Autodesk Fusion 360 part; units mm, degrees
(part 3 of 3)
  constraint parallel L321 L323
  constraint perpendicular L323 L324
  constraint perpendicular L322 L323
  constraint equal L289 L324
  constraint equal L290 L321
  constraint parallel L326 L328
  constraint perpendicular L327 L328
  constraint perpendicular L325 L328
  constraint collinear L27 L326
  constraint equal L324 L327
  constraint equal L321 L328
  constraint collinear L322 L325
  constraint parallel L330 L332
  constraint perpendicular L331 L332
  constraint perpendicular L329 L332
  constraint collinear L39 L332
  constraint collinear L325 L329
  constraint equal L328 L330
  constraint equal L325 L331
  constraint parallel L334 L336
  constraint perpendicular L335 L336
  constraint perpendicular L333 L336
  constraint equal L330 L336
  constraint equal L329 L333
  constraint collinear L329 L333
  constraint collinear L37 L334
  constraint parallel L350 L352
  constraint perpendicular L349 L352
  constraint perpendicular L351 L352
  constraint parallel L346 L347
  constraint perpendicular L346 L348
  constraint perpendicular L345 L346
  constraint equal L348 L349
  constraint equal L346 L350
  constraint collinear L345 L351
  constraint parallel L342 L343
  constraint perpendicular L341 L343
  constraint perpendicular L343 L344
  constraint collinear L344 L345
  constraint equal L342 L346
  constraint equal L341 L345
  constraint parallel L338 L340
  constraint perpendicular L337 L338
  constraint perpendicular L338 L339
  constraint equal L338 L342
  constraint equal L339 L344
  constraint parallel L366 L368
  constraint perpendicular L365 L368
  constraint perpendicular L367 L368
  constraint parallel L362 L363
  constraint perpendicular L362 L364
  constraint perpendicular L361 L362
  constraint equal L364 L365
  constraint equal L362 L366
  constraint collinear L361 L367
  constraint parallel L358 L359
  constraint perpendicular L357 L359
  constraint perpendicular L359 L360
  constraint collinear L360 L361
  constraint equal L358 L362
  constraint equal L357 L361
  constraint parallel L354 L356
  constraint perpendicular L353 L354
  constraint perpendicular L354 L355
  constraint equal L354 L358
  constraint equal L355 L360
  constraint collinear L355 L360
  constraint collinear L34 L340
  constraint collinear L32 L343
  constraint collinear L47 L347
  constraint collinear L45 L352
  constraint collinear L54 L356
  constraint collinear L349 L353
  constraint collinear L52 L359
  constraint collinear L58 L363
  constraint collinear L56 L368
  constraint equal L333 L337
  constraint equal L336 L338
  constraint collinear L337 L341
  constraint equal L351 L353
  constraint equal L350 L354
  constraint parallel L382 L383
  constraint perpendicular L383 L384
  constraint perpendicular L381 L383
  constraint parallel L377 L379
  constraint perpendicular L377 L380
  constraint perpendicular L377 L378
  constraint equal L380 L384
  constraint equal L377 L382
  constraint collinear L378 L381
  constraint parallel L374 L376
  constraint perpendicular L373 L374
  constraint perpendicular L374 L375
  constraint collinear L375 L378
  constraint equal L376 L377
  constraint equal L373 L378
  constraint parallel L369 L372
  constraint perpendicular L370 L372
  constraint perpendicular L371 L372
  constraint equal L372 L376
  constraint equal L371 L375
  constraint parallel L398 L400
  constraint perpendicular L397 L398
  constraint perpendicular L398 L399
  constraint parallel L394 L396
  constraint perpendicular L393 L394
  constraint perpendicular L394 L395
  constraint equal L393 L397
  constraint equal L394 L400
  constraint collinear L395 L399
  constraint parallel L389 L390
  constraint perpendicular L390 L392
  constraint perpendicular L390 L391
  constraint collinear L391 L395
  constraint equal L389 L394
  constraint equal L392 L395
  constraint parallel L386 L388
  constraint perpendicular L385 L386
  constraint perpendicular L386 L387
  constraint equal L386 L389
  constraint equal L387 L391
  constraint collinear L387 L391
  constraint collinear L384 L385
  constraint collinear L370 L373
  constraint equal L381 L385
  constraint equal L382 L386
  constraint equal L338 L372
  constraint equal L339 L370
  constraint collinear L42 L369
  constraint collinear L40 L374
  constraint collinear L30 L379
  constraint collinear L28 L383
  constraint collinear L50 L388
  constraint collinear L48 L390
  constraint collinear L62 L396
  constraint collinear L60 L398
  constraint parallel L414 L415
  constraint perpendicular L415 L416
  constraint perpendicular L413 L415
  constraint parallel L409 L411
  constraint perpendicular L409 L412
  constraint perpendicular L409 L410
  constraint equal L412 L416
  constraint equal L409 L414
  constraint collinear L410 L413
  constraint parallel L406 L408
  constraint perpendicular L405 L406
  constraint perpendicular L406 L407
  constraint collinear L407 L410
  constraint equal L408 L409
  constraint equal L405 L410
  constraint parallel L401 L404
  constraint perpendicular L402 L404
  constraint perpendicular L403 L404
  constraint equal L404 L408
  constraint equal L403 L407
  constraint parallel L430 L432
  constraint perpendicular L429 L430
  constraint perpendicular L430 L431
  constraint parallel L426 L428
  constraint perpendicular L425 L426
  constraint perpendicular L426 L427
  constraint equal L425 L429
  constraint equal L426 L432
  constraint collinear L427 L431
  constraint parallel L421 L422
  constraint perpendicular L422 L424
  constraint perpendicular L422 L423
  constraint collinear L423 L427
  constraint equal L421 L426
  constraint equal L424 L427
  constraint parallel L418 L420
  constraint perpendicular L417 L418
  constraint perpendicular L418 L419
  constraint equal L418 L421
  constraint equal L419 L423
  constraint collinear L419 L423
  constraint collinear L416 L417
  constraint collinear L402 L405
  constraint equal L413 L417
  constraint equal L414 L418
  constraint parallel L446 L447
  constraint perpendicular L447 L448
  constraint perpendicular L445 L447
  constraint parallel L441 L443
  constraint perpendicular L441 L444
  constraint perpendicular L441 L442
  constraint equal L444 L448
  constraint equal L441 L446
  constraint collinear L442 L445
  constraint parallel L438 L440
  constraint perpendicular L437 L438
  constraint perpendicular L438 L439
  constraint collinear L439 L442
  constraint equal L440 L441
  constraint equal L437 L442
  constraint parallel L433 L436
  constraint perpendicular L434 L436
  constraint perpendicular L435 L436
  constraint equal L436 L440
  constraint equal L435 L439
  constraint parallel L462 L464
  constraint perpendicular L461 L462
  constraint perpendicular L462 L463
  constraint parallel L458 L460
  constraint perpendicular L457 L458
  constraint perpendicular L458 L459
  constraint equal L457 L461
  constraint equal L458 L464
  constraint collinear L459 L463
  constraint parallel L453 L454
  constraint perpendicular L454 L456
  constraint perpendicular L454 L455
  constraint collinear L455 L459
  constraint equal L453 L458
  constraint equal L456 L459
  constraint parallel L450 L452
  constraint perpendicular L449 L450
  constraint perpendicular L450 L451
  constraint equal L450 L453
  constraint equal L451 L455
  constraint collinear L451 L455
  constraint collinear L448 L449
  constraint collinear L434 L437
  constraint equal L445 L449
  constraint equal L446 L450
  constraint parallel L478 L479
  constraint perpendicular L479 L480
  constraint perpendicular L477 L479
  constraint parallel L473 L475
  constraint perpendicular L473 L476
  constraint perpendicular L473 L474
  constraint equal L476 L480
  constraint equal L473 L478
  constraint collinear L474 L477
  constraint parallel L470 L472
  constraint perpendicular L469 L470
  constraint perpendicular L470 L471
  constraint collinear L471 L474
  constraint equal L472 L473
  constraint equal L469 L474
  constraint parallel L465 L468
  constraint perpendicular L466 L468
  constraint perpendicular L467 L468
  constraint equal L468 L472
  constraint equal L467 L471
  constraint parallel L494 L496
  constraint perpendicular L493 L494
  constraint perpendicular L494 L495
  constraint parallel L490 L492
  constraint perpendicular L489 L490
  constraint perpendicular L490 L491
  constraint equal L489 L493
  constraint equal L490 L496
  constraint collinear L491 L495
  constraint parallel L485 L486
  constraint perpendicular L486 L488
  constraint perpendicular L486 L487
  constraint collinear L487 L491
  constraint equal L485 L490
  constraint equal L488 L491
  constraint parallel L482 L484
  constraint perpendicular L481 L482
  constraint perpendicular L482 L483
  constraint equal L482 L485
  constraint equal L483 L487
  constraint collinear L483 L487
  constraint collinear L480 L481
  constraint collinear L466 L469
  constraint equal L477 L481
  constraint equal L478 L482
  constraint parallel L510 L511
  constraint perpendicular L511 L512
  constraint perpendicular L509 L511
  constraint parallel L505 L507
  constraint perpendicular L505 L508
  constraint perpendicular L505 L506
  constraint equal L508 L512
  constraint equal L505 L510
  constraint collinear L506 L509
  constraint parallel L502 L504
  constraint perpendicular L501 L502
  constraint perpendicular L502 L503
  constraint collinear L503 L506
  constraint equal L504 L505
  constraint equal L501 L506
  constraint parallel L497 L500
  constraint perpendicular L498 L500
  constraint perpendicular L499 L500
  constraint equal L500 L504
  constraint equal L499 L503
  constraint parallel L526 L528
  constraint perpendicular L525 L526
  constraint perpendicular L526 L527
  constraint parallel L522 L524
  constraint perpendicular L521 L522
  constraint perpendicular L522 L523
  constraint equal L521 L525
  constraint equal L522 L528
  constraint collinear L523 L527
  constraint parallel L517 L518
  constraint perpendicular L518 L520
  constraint perpendicular L518 L519
  constraint collinear L519 L523
  constraint equal L517 L522
  constraint equal L520 L523
  constraint parallel L514 L516
  constraint perpendicular L513 L514
  constraint perpendicular L514 L515
  constraint equal L514 L517
  constraint equal L515 L519
  constraint collinear L515 L519
  constraint collinear L512 L513
  constraint collinear L498 L501
  constraint equal L509 L513
  constraint equal L510 L514
  constraint collinear L17 L401
  constraint equal L372 L404
  constraint equal L371 L403
  constraint equal L402 L434
  constraint equal L404 L436
  constraint equal L436 L468
  constraint equal L435 L466
  constraint equal L467 L498
  constraint equal L468 L500
  constraint collinear L19 L406
  constraint collinear L10 L411
  constraint collinear L8 L415
  constraint collinear L3 L420
  constraint collinear L1 L422
  constraint collinear L221 L428
  constraint collinear L223 L430
  constraint collinear L187 L462
  constraint collinear L185 L460
  constraint collinear L7 L454
  constraint collinear L5 L452
  constraint collinear L183 L447
  constraint collinear L181 L443
  constraint collinear L13 L438
  constraint collinear L15 L433
  constraint collinear L195 L465
  constraint collinear L193 L470
  constraint collinear L205 L475
  constraint collinear L207 L479
  constraint collinear L214 L484
  constraint collinear L212 L486
  constraint collinear L176 L492
  constraint collinear L178 L494
  constraint collinear L197 L526
  constraint collinear L199 L524
  constraint collinear L191 L518
  constraint collinear L189 L516
  constraint collinear L211 L511
  constraint collinear L209 L507
  constraint collinear L203 L502
  constraint collinear L201 L497
  constraint parallel L533 L535
  constraint perpendicular L533 L536
  constraint perpendicular L533 L534
  constraint parallel L529 L532
  constraint perpendicular L529 L530
  constraint perpendicular L529 L531
  constraint equal L530 L536
  constraint equal L529 L535
  constraint collinear L531 L534
  constraint parallel L541 L543
  constraint perpendicular L541 L544
  constraint perpendicular L541 L542
  constraint parallel L537 L540
  constraint perpendicular L537 L538
  constraint perpendicular L537 L539
  constraint equal L538 L544
  constraint equal L537 L543
  constraint collinear L539 L542
  constraint parallel L549 L551
  constraint perpendicular L549 L552
  constraint perpendicular L549 L550
  constraint parallel L545 L548
  constraint perpendicular L545 L546
  constraint perpendicular L545 L547
  constraint equal L546 L552
  constraint equal L545 L551
  constraint collinear L547 L550
  constraint collinear L525 L546
  constraint collinear L216 L548
  constraint collinear L218 L549
  constraint equal L528 L545
  constraint equal L527 L547
  constraint collinear L20 L540
  constraint collinear L22 L541
  constraint collinear L493 L538
  constraint equal L496 L537
  constraint equal L495 L539
  constraint collinear L225 L532
  constraint collinear L461 L530
  constraint collinear L227 L533
  constraint equal L463 L531
  constraint equal L464 L529
  constraint parallel L557 L559
  constraint perpendicular L557 L560
  constraint perpendicular L557 L558
  constraint parallel L553 L556
  constraint perpendicular L553 L554
  constraint perpendicular L553 L555
  constraint equal L554 L560
  constraint equal L553 L559
  constraint collinear L555 L558
  constraint collinear L102 L556
  constraint collinear L100 L557
  constraint equal L432 L553
  constraint equal L399 L555
  constraint perpendicular L119 L561
  constraint perpendicular L114 L562
  constraint coincident L109 L563.start
  constraint perpendicular L109 L563
  constraint perpendicular L108 L564
  constraint coincident L109 L565.end
  constraint perpendicular L109 L565
  constraint perpendicular L126 L567
  constraint coincident L137 L569.start
  constraint perpendicular L137 L569
  constraint perpendicular L569 L570
  constraint coincident L137 L571.end
  constraint perpendicular L137 L571
  constraint equal L565 L569
  constraint equal L564 L570
  constraint perpendicular L168 L573
  constraint perpendicular L173 L574
  constraint perpendicular L155 L576
  constraint coincident L142 L577.start
  constraint perpendicular L142 L577
  constraint perpendicular L577 L578
  constraint coincident L142 L579.end
  constraint perpendicular L142 L579
  constraint equal L570 L578
  constraint equal L571 L577
  constraint coincident L150 L581.start
  constraint perpendicular L150 L581
  constraint perpendicular L581 L582
  constraint coincident L150 L583.end
  constraint perpendicular L150 L583
  constraint equal L577 L583
  constraint equal L578 L582
  constraint perpendicular L82 L586
  constraint perpendicular L94 L587
  constraint coincident L69 L589.start
  constraint perpendicular L69 L589
  constraint perpendicular L589 L590
  constraint coincident L69 L591.end
  constraint perpendicular L69 L591
  constraint equal L578 L590
  constraint equal L579 L591
  constraint coincident L77 L593.start
  constraint perpendicular L77 L593
  constraint perpendicular L593 L594
  constraint coincident L77 L595.end
  constraint perpendicular L77 L595
  constraint equal L578 L594
  constraint equal L591 L595
  constraint collinear L598 L601
  constraint horizontal L602
  constraint vertical L603
  constraint collinear L603 L605
  constraint horizontal L597
  constraint horizontal L607
  constraint vertical L608
  constraint horizontal L609
  constraint vertical L610
  constraint horizontal L611
  constraint vertical L612
  constraint horizontal L613
  constraint vertical L614
  constraint collinear L607 L615
  constraint collinear L611 L616
  constraint equal L609 L613
  constraint equal L608 L614
  constraint equal L589 L610
  constraint equal L590 L609
  constraint perpendicular L568 L617
  constraint coincident L132 L618.end
  constraint perpendicular L125 L618
  constraint coincident L114 L619.end
  constraint perpendicular L114 L619
  constraint perpendicular L619 L620
  constraint collinear L121 L619
  constraint collinear L562 L567
  constraint collinear L120 L561
  constraint collinear L126 L568
  constraint parallel L623 L624
  constraint perpendicular L621 L623
  constraint perpendicular L622 L623
  constraint collinear L105 L623
  constraint equal L560 L622
  constraint equal L559 L624
  constraint parallel L627 L628
  constraint perpendicular L625 L627
  constraint perpendicular L626 L627
  constraint collinear L146 L627
  constraint equal L624 L628
  constraint equal L621 L626
  constraint coincident L173 L629.end
  constraint perpendicular L574 L629
  constraint coincident L155 L630.end
  constraint perpendicular L155 L630
  constraint perpendicular L576 L631
  constraint collinear L166 L630
  constraint collinear L574 L576
  constraint collinear L161 L575
  constraint collinear L167 L573
  constraint coincident L64 L633.end
  constraint perpendicular L587 L633
  constraint coincident L82 L634.end
  constraint perpendicular L82 L634
  constraint perpendicular L586 L635
  constraint perpendicular L585 L636
  constraint collinear L93 L634
  constraint collinear L586 L587
  constraint collinear L88 L585
  constraint collinear L94 L588
  constraint parallel L639 L640
  constraint perpendicular L637 L639
  constraint perpendicular L638 L639
  constraint collinear L73 L639
  constraint equal L366 L640
  constraint equal L365 L638
  constraint coincident L600 L641.end
  constraint perpendicular L597 L641
  constraint coincident L604 L642.end
  constraint perpendicular L604 L642
  constraint perpendicular L602 L643
  constraint perpendicular L598 L644
  constraint collinear L597 L602
  constraint collinear L642 L645
  constraint horizontal L647
  constraint vertical L648
  constraint horizontal L646
  constraint vertical L649
  constraint collinear L646 L650
  constraint collinear L283 L649
  constraint equal L281 L648
  constraint collinear L281 L648
  measures "d504" distance of L237 L239
  measures "d508" distance of L243 L248
  measures "d510" distance of L246 L249
  measures "d511" distance of L17 L231
  measures "d514" distance of L229 L233
  measures "d515" distance of L228 L232
  measures "d516" distance of L230 L231
  measures "d517" distance of L238 L240
  measures "d518" distance of L238 L246
  measures "d519" distance of L244 L247
  measures "d520" distance of L245 L251
  measures "d563" distance of L254 L256
  measures "d564" distance of L252.end L253.end
  measures "d565" distance of L253 L255
  measures "d566" distance of L257 L258
  measures "d567" distance of L254 L263
  measures "d568" distance of L271 L275
  measures "d569" distance of L270 L276
  measures "d570" distance of L271.end L281.end
  measures "d571" distance of L281.end L289.end
  measures "d572" distance of L296 L309
  measures "d614" distance of L24 L324
  measures "d638" distance of L33 L339
  measures "d639" distance of L43 L370
  measures "d640" distance of L18 L402
  measures "d641" distance of L12 L434
  measures "d642" distance of L192 L466
  measures "d643" distance of L202 L498
  measures "d644" distance of L103 L554
  measures "d674" distance of L563.end L564.end
  measures "d676" distance of L108.end L565
  measures "d678" distance of L564 L566
  measures "d679" distance of L137.end L569.start
  measures "d680" distance of L141 L579
  measures "d681" distance of L149 L583
  measures "d682" distance of L68 L589
  measures "d683" distance of L78 L593
  measures "d684" distance of L610 L615.end
  measures "d685" distance of L612 L616.start
  measures "d687" distance of L115 L562
  measures "d688" distance of L562 L617
  measures "d689" distance of L106 L622
  measures "d690" distance of L145 L625.start
  measures "d691" distance of L576 L632
  measures "d692" distance of L156 L576
  measures "d693" distance of L83 L586
  measures "d694" distance of L586 L636
  measures "d695" distance of L72 L637
  measures "d696" distance of L597 L599
  measures "d697" distance of L597 L644
extrude "Rahmen Rechts" add sketch "Skizze4" along normal up to surface separate body contours L228 L229 A0 L230 A1 L237 L238 A2 end surface through (0, 80, 16.2816) normal (0, 0.043619, -0.999048) offset 0 makes body 3
extrude "Rahmen Mitte" add sketch "Skizze4" along normal up to surface separate body contours L238 L247 L248 L251 end surface through (0, 80, 16.2816) normal (0, 0.043619, -0.999048) offset 0 makes body 4
fillet "Abrundung1" radius 2 7 edges at (-104.3906, 28.0489, 0) (-163.9894, 43.7866, 0) (-62.3093, 1.7662, 0) (-41.6839, 0, 0) (-176.2508, 102.7417, 0) (-100.1502, 146.1161, 0) (-32.4236, 134.2339, 0) on bodies 1 2
fillet "Abrundung1" radius 2 2 edges at (0, 0, 0) (0, 134.175, 0) on bodies 1 2
ref_plane "Arbeitsebene2" through (0, 0, 10.7) normal (0, 0, 1) x (1, 0, 0)
sketch "Skizze6" plane through (0, 0, 10.7) normal (0, 0, 1) x (1, 0, 0)
  line L0 (-163.5373, 153.5359) -> (-33.425, 130.5936)
  line L1 (-164.3485, 154.6944) -> (-32.425, 131.4327)
  line L2 (-163.5373, 153.5359) -> (-181.6767, 50.6624)
  line L3 (-182.8351, 49.8513) -> (-164.3485, 154.6944)
  line L4 (-181.6767, 50.6624) -> (-141.3734, 43.5559)
  line L5 (-141.5471, 42.5711) -> (-182.8351, 49.8513)
  line L6 (-141.3734, 43.5559) -> (-141.5471, 42.5711) construction
  line L7 (-52.2928, 3.7) -> (-33.425, 3.7)
  arc A0 (-68.7394, 9.6861) -> (-141.3734, 43.5559) centre (-168.2583, -108.916) ccw
  arc A1 (-68.7394, 9.6861) -> (-52.2928, 3.7) centre (-52.2928, 29.2863) ccw
  line L8 (0, 130.475) -> (0, 128.475) construction
  line L9 (0, 128.475) -> (-11, 128.475)
  line L10 (-11, 128.475) -> (-11, 130.475)
  line L11 (0, 128.475) -> (11, 128.475)
  line L12 (11, 128.475) -> (11, 130.475)
  line L13 (-52.2928, 3.7) -> (-52.2928, 2.7) construction
  line L14 (-32.425, 2.7) -> (-52.2928, 2.7) construction
  line L15 (-68.7394, 9.6861) -> (-69.3822, 8.92) construction
  line L16 (-58.4402, 21.9601) -> (-59.4205, 20.7919) construction
  line L17 (-33.425, 3.7) -> (-33.425, 130.5936)
  line L18 (-32.425, 131.4327) -> (-32.425, 2.7)
  line L19 (28.725, 3.7) -> (-28.725, 3.7)
  line L20 (-28.725, 3.7) -> (-28.725, 130.475)
  line L21 (-28.725, 130.475) -> (28.725, 130.475)
  line L22 (28.725, 130.475) -> (28.725, 3.7)
  line L23 (29.725, 131.475) -> (29.725, 2.7)
  line L24 (29.725, 2.7) -> (-29.725, 2.7)
  line L25 (-29.725, 2.7) -> (-29.725, 131.475)
  line L26 (-29.725, 131.475) -> (29.725, 131.475)
  line L27 (0, 1.75) -> (0, 22.5)
  point P0 (-52.2928, 2.7)
  point P1 (-69.3822, 8.92)
  dimension "d489" = 2
  dimension "d490" = 11
  dimension "d491" = 11
  dimension "d525" = 1
  dimension "d526" = 1
  dimension "d527" = 1
  dimension "d528" = 1
  dimension "d529" = 1
  dimension "d530" = 1
  dimension "d531" = 1
  dimension "d532" = 1
  dimension "d533" = 1
  constraint parallel L0 L1
  constraint perpendicular L0 L2
  constraint perpendicular L2 L4
  constraint coincident L5.start L6.end
  constraint perpendicular L4 L6
  constraint tangent L4 A0
  constraint tangent A0 A1
  constraint vertical L8
  constraint perpendicular L8 L9
  constraint perpendicular L9 L10
  constraint perpendicular L8 L11
  constraint perpendicular L11 L12
  constraint horizontal L7
  constraint perpendicular L7 L13
  constraint coincident P0 L13.end
  constraint tangent L7 A1
  constraint coincident P1 L15.end
  constraint collinear L15 L16
  constraint parallel L17 L18
  constraint horizontal L19
  constraint vertical L20
  constraint horizontal L21
  constraint vertical L22
  constraint coincident L12.end L21
  constraint coincident L8.start L21
  constraint coincident L10.end L21
  constraint collinear L8 L27
  measures "d489" distance of L8.start L8.end
  measures "d490" distance of L8.end L9.end
  measures "d491" distance of L8.end L11.end
  measures "d525" distance of L7 L14
  measures "d526" distance of L4 L5
  measures "d527" distance of L2 L3
  measures "d528" distance of L0 L1
  measures "d529" distance of L17 L18
  measures "d530" distance of L22 L23
  measures "d531" distance of L19 L24
  measures "d532" distance of L20 L25
  measures "d533" distance of L21 L26
extrude "Bodenplatte Rechts" add sketch "Skizze6" along normal up to surface separate body contours L0 L2 L4 L7 A0 A1 L17 end surface through (0, 80, 16.2816) normal (0, 0.043619, -0.999048) offset 0 makes body 5
extrude "Bodenplatte Mitte" add sketch "Skizze6" along normal up to surface separate body contours L9 L10 L11 L12 L19 L20 L21 L22 | L9 L10 L11 L12 L21 end surface through (0, 80, 16.2816) normal (0, 0.043619, -0.999048) offset 0 makes body 6
extrude "Lasche an Bodenplatte" add sketch "Skizze6" against normal blind 6 contours L9 L10 L11 L12 L21 bodies 6
ref_plane "Arbeitsebene3" through (-107.5508, 78.7357, 13.5239) normal (0, -0.043619, 0.999048) x (1, 0, 0)
sketch "Skizze7" plane through (0, 78.9574, 13.5335) normal (0, -0.043619, 0.999048) x (1, 0, 0)
  line L0 (11, 49.6846) -> (-11, 49.6846)
  line L1 (0, -77.7242) -> (0, -56.994)
  line L2 (11, 49.6846) -> (11, -2.3154)
  line L3 (11, -2.3154) -> (-11, -2.3154)
  line L4 (-11, -2.3154) -> (-11, 49.6846)
  circle A0 centre (-5.7, 0.1846) radius 0.75
  circle A1 centre (5.7, 0.1846) radius 0.75
  circle A2 centre (5.7, 47.1846) radius 0.75
  circle A3 centre (-5.7, 47.1846) radius 0.75
  line L5 (28.725, 51.6846) -> (-28.725, 51.6846)
  line L6 (-13, -2.3154) -> (-13, 51.6846)
  line L7 (-13, 51.6846) -> (-28.725, 51.6846)
  line L8 (-28.725, 51.6846) -> (-28.725, -75.3094)
  line L9 (-28.725, -75.3094) -> (28.725, -75.3094)
  line L10 (28.725, -75.3094) -> (28.725, 51.6846)
  line L11 (28.725, 51.6846) -> (13, 51.6846)
  line L12 (13, 51.6846) -> (13, -2.3154)
  line L13 (11, -4.3154) -> (-11, -4.3154)
  arc A4 (11, -4.3154) -> (13, -2.3154) centre (11, -2.3154) ccw
  arc A5 (-13, -2.3154) -> (-11, -4.3154) centre (-11, -2.3154) ccw
  line L14 (-28.725, -75.3094) -> (-28.725, 51.345)
  line L15 (28.725, 51.345) -> (28.725, -75.3094)
  line L16 (28.725, -75.3094) -> (-28.725, -75.3094)
  line L17 (11, 49.6846) -> (13, 49.6846)
  line L18 (-11, 49.6846) -> (-13, 49.6846)
  dimension "d458" = 52
  dimension "d460" = 1.5
  dimension "d461" = 1.5
  dimension "d462" = 2.5
  dimension "d463" = 2.5
  dimension "d464" = 5.3
  dimension "d465" = 5.3
  dimension "d466" = 11.4
  dimension "d467" = 1.5
  dimension "d468" = 1.5
  dimension "d469" = 2.5
  dimension "d470" = 2.5
  dimension "d471" = 5.3
  dimension "d472" = 5.3
  dimension "d473" = 11.4
  dimension "d536" = 2
  dimension "d537" = 11
  dimension "d538" = 11
  dimension "d704" = 2
  constraint horizontal L0
  constraint perpendicular L0 L2
  constraint perpendicular L2 L3
  constraint perpendicular L0 L4
  constraint perpendicular L5 L6
  constraint perpendicular L6 L7
  constraint perpendicular L8 L9
  constraint perpendicular L5 L10
  constraint parallel L5 L11
  constraint perpendicular L3 L12
  constraint perpendicular L4 L13
  constraint coincident L2.end L3.start
  constraint coincident L3 L6.start
  constraint coincident L4 L13.end
  constraint coincident L2 L13.start
  constraint coincident L3 L12.end
  constraint tangent L6 A5
  constraint tangent L13 A5
  constraint collinear L5 L7
  constraint collinear L5 L11
  constraint collinear L8 L14
  constraint collinear L10 L15
  constraint collinear L9 L16
  constraint coincident L12 L17.end
  constraint perpendicular L12 L17
  constraint coincident L6 L18.end
  constraint perpendicular L6 L18
  measures "d458" distance of L0.start L2.end
  measures "d460" diameter of A0
  measures "d461" diameter of A1
  measures "d462" distance of L3 A1.centre
  measures "d463" distance of L3 A0.centre
  measures "d464" distance of L4 A0.centre
  measures "d465" distance of L2 A1.centre
  measures "d466" distance of A0.centre A1.centre
  measures "d467" diameter of A2
  measures "d468" diameter of A3
  measures "d469" distance of L0 A3.centre
  measures "d470" distance of L0 A2.centre
  measures "d471" distance of L4 A3.centre
  measures "d472" distance of L2 A2.centre
  measures "d473" distance of A2.centre A3.centre
  measures "d536" distance of L0 L5
  measures "d537" distance of L1 L2
  measures "d538" distance of L1 L4
  measures "d704" distance of L3 L13
extrude "Ausschnitt Controller (1)" cut sketch "Skizze7" against normal through all contours L0 L2 L3 L4 | L2 L3 L4 L6 L12 L13 A4 A5 L17 L18 | L5 L6 L7 L8 L9 L10 L11 L12 L13 A4 A5 L14 L15 L16 | A0 | A1 | A2 | A3 bodies 6
extrude "Stifte Controller" add sketch "Skizze7" against normal blind 1.5 contours L2 L3 L4 L6 L12 L13 A4 A5 L17 L18 | A0 | A1 | A2 | A3 bodies 6
extrude "Extrusion27" add sketch "Skizze1" along normal up to surface from surface at 10.7 contours A3 | A4 | A5 | A6 | A7 | A8 | A9 | A10 | A11 | A12 | A13 | A14 | A39 | A40 | A41 | A42 | A43 | A44 | A57 | A58 | A59 | A60 | A61 | A62 end surface through (0, 78.9574, 13.5335) normal (0, 0.043619, -0.999048) offset 0 bodies 6
sketch "Skizze8" plane through (0, 129.0342, 5.6338) normal (0, -0.999048, -0.043619) x (1, 0, 0)
  line L0 (11, 10.0766) -> (-11, 10.0766)
  line L1 (4.5, 5.0766) -> (-4.5, 5.0766)
  line L2 (-4.5, 5.0766) -> (-4.5, 9.0766)
  line L3 (-4.5, 9.0766) -> (4.5, 9.0766)
  line L4 (4.5, 9.0766) -> (4.5, 5.0766)
  line L5 (7, 2.0766) -> (-7, 2.0766)
  line L6 (-7, 2.0766) -> (-7, 13.0766)
  line L7 (7, 2.0766) -> (7, 13.0766)
  line L8 (7, 13.0766) -> (-7, 13.0766)
  line L9 (-11, -0.9346) -> (11, -0.9346)
  line L10 (11, -0.9346) -> (11, 5.0711)
  line L11 (-11, 5.0711) -> (-11, -0.9346)
  line L12 (11, 5.0711) -> (13, 5.0711)
  line L13 (13, 5.0711) -> (13, 8.5766)
  line L14 (-13, 8.5766) -> (-13, 5.0711)
  line L15 (-13, 5.0711) -> (-11, 5.0711)
  line L16 (-11, 8.5766) -> (-13, 8.5766)
  line L17 (13, 8.5766) -> (11, 8.5766)
  line L18 (11, 8.5766) -> (11, 10.0766)
  line L19 (-11, 10.0766) -> (-11, 8.5766)
  line L20 (11, 5.0711) -> (11, 8.5766)
  line L21 (-11, 5.0711) -> (-11, 8.5766)
  line L22 (13, 5.0711) -> (13, 4.0711)
  line L23 (13, 4.0711) -> (11, 4.0711)
  line L24 (-13, 5.0711) -> (-13, 4.0711)
  line L25 (-13, 4.0711) -> (-11, 4.0711)
  dimension "d477" = 5
  dimension "d478" = 1
  dimension "d485" = 8
  dimension "d486" = 14
  dimension "d487" = 11
  dimension "d542" = 2.5
  dimension "d576" = 6.5
  dimension "d714" = 9
  dimension "d715" = 4
  dimension "d716" = 2.5
  dimension "d717" = 1
  dimension "d718" = 1
  constraint horizontal L1
  constraint vertical L2
  constraint horizontal L3
  constraint vertical L4
  constraint horizontal L5
  constraint perpendicular L0 L6
  constraint perpendicular L0 L7
  constraint horizontal L8
  constraint coincident L10.end L12.start
  constraint coincident L17.end L18.start
  constraint coincident L11.start L15.end
  constraint coincident L16.start L19.end
  constraint coincident L12.end L13.start
  constraint perpendicular L12 L22
  constraint coincident L10 L23.end
  constraint perpendicular L10 L23
  constraint coincident L14.end L15.start
  constraint perpendicular L15 L24
  constraint coincident L11 L25.end
  constraint perpendicular L11 L25
  measures "d477" distance of L0 L1
  measures "d478" distance of L0 L3
  measures "d485" distance of L0 L5
  measures "d486" distance of L5.start L5.end
  measures "d487" distance of L5 L8
  measures "d542" distance of L2 L6
  measures "d576" horizontal distance of L1.end L9.start
  measures "d714" distance of L1.start L1.end
  measures "d715" distance of L6 L11
  measures "d716" distance of L4 L7
  measures "d717" distance of L12.end L22.end
  measures "d718" distance of L14.end L24.end
extrude "Öffnung in Grundplatte" cut sketch "Skizze8" against normal through all contours L12 L13 L17 L20 | L10 L12 L22 L23 | L14 L15 L16 L21 | L11 L15 L24 L25 | L1 L2 L3 L4 bodies 6
extrude "Öffnug in Rahmen" cut sketch "Skizze8" against normal through all contours L0 L5 L6 L7 | L0 L6 L7 L8 | L1 L2 L3 L4 bodies 4
extrude "Stehhülsen" add sketch "Skizze1" along normal blind 10.7 contours A3 | A4 | A5 | A6 | A7 | A8 | A9 | A10 | A11 | A12 | A13 | A14 | A15 | A16 | A17 | A18 | A19 | A20 | A21 | A22 | A23 | A24 | A25 | A26 | A27 | A28 | A29 | A30 | A31 | A32 | A33 | A34 | A35 | A36 | A37 | A38 bodies 1 2 3 4
extrude "Bohrungen" cut sketch "Skizze1" along normal through all contours A3 | A5 | A7 | A9 | A11 | A13 | A15 | A17 | A19 | A21 | A23 | A25 | A27 | A29 | A31 | A33 | A35 | A37 | A39 | A40 | A41 | A42 | A43 | A44 | A45 | A46 | A47 | A48 | A49 | A50 | A51 | A52 | A53 | A54 | A55 | A56 bodies 5 6
extrude "Senkungen" cut sketch "Skizze1" along normal through all from surface at 12.2 contours A4 | A6 | A8 | A10 | A12 | A14 | A16 | A18 | A20 | A22 | A24 | A26 | A28 | A30 | A32 | A34 | A36 | A38 bodies 5 6
extrude "Kerben" cut sketch "Skizze4" against normal blind 1.4 contours L3 L417 L418 L419 L420 | L1 L421 L422 L423 L424 | L7 L453 L454 L455 L456 | L5 L449 L450 L451 L452 | L8 L413 L414 L415 L416 | L10 L409 L410 L411 L412 | L15 L433 L434 L435 L436 | L13 L437 L438 L439 L440 | L19 L405 L406 L407 L408 | L17 L401 L402 L403 L404 | L20 L537 L538 L539 L540 | L22 L541 L542 L543 L544 | L27 L325 L326 L327 L328 | L25 L321 L322 L323 L324 | L28 L381 L382 L383 L384 | L30 L377 L378 L379 L380 | L32 L341 L342 L343 L344 | L34 L337 L338 L339 L340 | L39 L329 L330 L331 L332 | L37 L333 L334 L335 L336 | L40 L373 L374 L375 L376 | L42 L369 L370 L371 L372 | L47 L345 L346 L347 L348 | L45 L349 L350 L351 L352 | L48 L389 L390 L391 L392 | L50 L385 L386 L387 L388 | L52 L357 L358 L359 L360 | L54 L353 L354 L355 L356 | L56 L365 L366 L367 L368 | L58 L361 L362 L363 L364 | L60 L397 L398 L399 L400 | L62 L393 L394 L395 L396 | L83 L84 L85 L86 L87 L88 L89 L90 L91 L92 L93 L94 L95 L96 L97 L98 L99 L585 L586 L587 L588 L633 L634 L635 L636 | L69 L589 L590 L591 L592 | L77 L593 L594 L595 L596 | L73 L637 L638 L639 L640 | L100 L557 L558 L559 L560 | L102 L553 L554 L555 L556 | L105 L621 L622 L623 L624 | L137 L569 L570 L571 L572 | L109 L563 L564 L565 L566 | L115 L116 L117 L118 L119 L120 L121 L122 L123 L124 L125 L126 L127 L128 L129 L130 L131 L561 L562 L567 L568 L617 L618 L619 L620 | L142 L577 L578 L579 L580 | L156 L157 L158 L159 L160 L161 L162 L163 L164 L165 L166 L167 L168 L169 L170 L171 L172 L573 L574 L575 L576 L629 L630 L631 L632 | L146 L625 L626 L627 L628 | L150 L581 L582 L583 L584 | L176 L489 L490 L491 L492 | L178 L493 L494 L495 L496 | L183 L445 L446 L447 L448 | L181 L441 L442 L443 L444 | L187 L461 L462 L463 L464 | L185 L457 L458 L459 L460 | L191 L517 L518 L519 L520 | L189 L513 L514 L515 L516 | L195 L465 L466 L467 L468 | L193 L469 L470 L471 L472 | L199 L521 L522 L523 L524 | L197 L525 L526 L527 L528 | L203 L501 L502 L503 L504 | L201 L497 L498 L499 L500 | L207 L477 L478 L479 L480 | L205 L473 L474 L475 L476 | L211 L509 L510 L511 L512 | L209 L505 L506 L507 L508 | L212 L485 L486 L487 L488 | L214 L481 L482 L483 L484 | L216 L545 L546 L547 L548 | L218 L549 L550 L551 L552 | L223 L429 L430 L431 L432 | L221 L425 L426 L427 L428 | L227 L533 L534 L535 L536 | L225 L529 L530 L531 L532 | L252 L253 L254 L257 | L258 L259 L260 L261 | L262 L263 L264 L265 | L266 L267 L268 L269 | L270 L271 L272 L273 L274 | L276 L277 L278 L279 | L280 L281 L282 L283 | L284 L285 L286 L287 | L288 L289 L290 L291 | L292 L293 L294 L295 | L296 L297 L298 L299 L300 | L301 L302 L303 L304 | L305 L306 L307 L308 | L309 L310 L311 L312 | L313 L314 L315 L316 | L317 L318 L319 L320 | L597 L598 L600 L602 L603 L604 L641 L642 L643 L644 L645 | L607 L608 L609 L610 L615 | L611 L612 L613 L614 L616 | L646 L647 L648 L649 L650 bodies 1 2
sketch "Skizze9" plane through (-32.425, 0, 0) normal (-1, 0, 0) x (0, -1, 0)
  line L0 (-2.7, 12.9066) -> (-131.4327, 18.5272)
  line L1 (-131.4327, 18.5272) -> (-131.4327, 2.7)
  line L2 (-131.4327, 2.7) -> (-2.7, 2.7)
  line L3 (-2.7, 2.7) -> (-2.7, 12.9066)
  circle A0 centre (-104.8827, 10.034) radius 1.25
  circle A1 centre (-66.225, 9.1901) radius 1.25
  circle A2 centre (-28.125, 8.3584) radius 1.25
  line L4 (-2.7, 7.8033) -> (-131.4327, 10.6136) construction
  circle A3 centre (-85.5538, 9.6121) radius 2.25
  circle A4 centre (-47.175, 8.7742) radius 2.25
  point P0 (-131.4327, 10.6136)
  point P1 (-2.7, 7.8033)
  dimension "d622" = 2.5
  dimension "d624" = 2.5
  dimension "d625" = 2.5
  dimension "d628" = 63.525
  dimension "d629" = 25.425
  dimension "d630" = 26.55
  dimension "d632" = 4.5
  dimension "d633" = 4.5
  dimension "d634" = 19.05
  dimension "d635" = 38.1
  dimension "d636" = 38.6577
  dimension "d637" = 19.3288
  constraint midpoint L1 P0
  constraint midpoint L3 P1
  constraint coincident P1 L4.start
  constraint coincident P0 L4.end
  constraint coincident A0.centre L4
  constraint coincident A1.centre L4
  constraint coincident A2.centre L4
  constraint coincident L4 A3.centre
  constraint coincident L4 A4.centre
  measures "d622" diameter of A0
  measures "d624" diameter of A1
  measures "d625" diameter of A2
  measures "d628" distance of L3 A1.centre
  measures "d629" distance of L3 A2.centre
  measures "d630" distance of L1 A0.centre
  measures "d632" diameter of A3
  measures "d633" diameter of A4
  measures "d634" horizontal distance of A2.centre A4.centre
  measures "d635" horizontal distance of A1.centre A2.centre
  measures "d636" horizontal distance of A0.centre A1.centre
  measures "d637" horizontal distance of A0.centre A3.centre
extrude "Verbindungslöcher (1)" cut sketch "Skizze9" against normal through all contours A0 | A1 | A2 | A3 | A4 bodies 3 4
mirror "Spiegeln1" about plane through (0, 0, 0) normal (1, 0, 0) of bodies 1 5 3 makes body 7 at (44.8497, 7.2478, 2.7) makes body 8 at (43.1742, 69.1197, 10.7) makes body 9 at (122.2797, 150.0181, 13.6789)
equation "Lochabstand = 19.05 mm"
equation "Lochgröße = 14 mm"
equation "Stegbreite = Lochabstand - Lochgröße"
equation "Plattenstärke = 2.7 mm"
equation "Senkung = Bodendicke / 2"
equation "Wandstärke = 3 mm" comment "Nicht nutzen. Änderungen dieses Parameters verursachen Fehler!"
equation "Gehäusehöhe = 17.6 mm + Bodendicke"
equation "Bohrung = 2.5 mm"
equation "Schraubenkopf = 4.5 mm"
equation "Kerbtiefe = 1 mm"
equation "Kerblänge = 5 mm"
equation "Kerbhöhe = 1.4 mm"
equation "Bodendicke = Plattenstärke"
equation "d2 = Lochgröße"
equation "d3 = Lochgröße"
equation "d6 = Lochgröße"
equation "d7 = Lochgröße"
equation "d9 = Lochgröße"
equation "d10 = Lochgröße"
equation "d11 = Lochgröße"
equation "d12 = Lochgröße"
equation "d13 = Stegbreite"
equation "d14 = Lochgröße"
equation "d15 = Lochgröße"
equation "d16 = Lochgröße"
equation "d17 = Lochgröße"
equation "d128 = Lochgröße"
equation "d129 = Lochgröße"
equation "d130 = Lochgröße"
equation "d131 = Lochgröße"
equation "d132 = Stegbreite"
equation "d133 = Stegbreite"
equation "d134 = Stegbreite"
equation "d135 = Stegbreite"
equation "d136 = Stegbreite"
equation "d137 = Stegbreite"
equation "d138 = Lochgröße"
equation "d139 = Lochgröße"
equation "d140 = Stegbreite"
equation "d142 = Lochgröße"
equation "d143 = Lochgröße"
equation "d144 = Lochgröße"
equation "d145 = Lochgröße"
equation "d146 = Lochgröße"
equation "d147 = Lochgröße"
equation "d148 = Lochgröße"
equation "d149 = Lochgröße"
equation "d150 = Stegbreite"
equation "d151 = Lochgröße"
equation "d152 = Lochgröße"
equation "d153 = Lochgröße"
equation "d154 = Lochgröße"
equation "d155 = Lochgröße"
equation "d156 = Lochgröße"
equation "d157 = Lochgröße"
equation "d158 = Lochgröße"
equation "d159 = Stegbreite"
equation "d160 = Stegbreite"
equation "d161 = Stegbreite"
equation "d162 = Stegbreite"
equation "d163 = Stegbreite"
equation "d164 = Stegbreite"
equation "d165 = Lochgröße"
equation "d166 = Lochgröße"
equation "d167 = Stegbreite"
equation "d169 = Stegbreite"
equation "d170 = Lochgröße"
equation "d171 = Lochgröße"
equation "d172 = Stegbreite"
equation "d176 = Lochgröße"
equation "d177 = Lochgröße"
equation "d180 = Lochgröße"
equation "d181 = Lochgröße"
equation "d191 = Stegbreite"
equation "d201 = Lochgröße"
equation "d202 = Lochgröße"
equation "d203 = Lochgröße"
equation "d204 = Lochgröße"
equation "d205 = Lochgröße"
equation "d206 = Lochgröße"
equation "d207 = Lochgröße"
equation "d208 = Lochgröße"
equation "d209 = Stegbreite"
equation "d210 = Lochgröße"
equation "d211 = Lochgröße"
equation "d212 = Lochgröße"
equation "d213 = Lochgröße"
equation "d214 = Lochgröße"
equation "d215 = Lochgröße"
equation "d218 = Stegbreite"
equation "d219 = Stegbreite"
equation "d220 = Stegbreite"
equation "d221 = Stegbreite"
equation "d222 = Stegbreite"
equation "d224 = Lochgröße"
equation "d225 = Lochgröße"
equation "d226 = Stegbreite"
equation "d227 = Stegbreite"
equation "d232 = Stegbreite"
equation "d258 = 1.5 * Stegbreite + Lochgröße / 2"
equation "d280 = Lochgröße"
equation "d281 = Lochgröße"
equation "d282 = Lochgröße"
equation "d283 = Lochgröße"
equation "d284 = Stegbreite"
equation "d285 = Stegbreite"
equation "d286 = Stegbreite / 2"
equation "d287 = Lochgröße"
equation "d288 = Lochgröße"
equation "d289 = Lochgröße"
equation "d290 = Lochgröße"
equation "d291 = Stegbreite"
equation "d292 = Lochgröße"
equation "d293 = Lochgröße"
equation "d294 = Stegbreite"
equation "d295 = Lochgröße"
equation "d296 = Lochgröße"
equation "d297 = Lochgröße"
equation "d298 = Lochgröße"
equation "d300 = Lochgröße"
equation "d301 = Lochgröße"
equation "d303 = Stegbreite"
equation "d305 = Stegbreite"
equation "d306 = Lochgröße"
equation "d307 = Lochgröße"
equation "d409 = -7 mm + 18.55 mm"
equation "d412 = d409"
equation "d416 = d409"
equation "d420 = d409"
equation "d423 = Stegbreite / 2 + Wandstärke + 1 mm"
equation "d424 = d423"
equation "d426 = Plattenstärke"
equation "d444 = Plattenstärke + Stützhöhe"
equation "d451 = Plattenstärke + 8 mm + Bodendicke"
equation "d454 = -Bodendicke"
equation "d496 = ( Stegbreite + Wandstärke ) / 2 + 1 mm"
equation "d497 = d496"
equation "d498 = d496"
equation "d499 = d423 + d235"
equation "d501 = Plattenstärke"
equation "d504 = Plattenstärke"
equation "d508 = Plattenstärke"
equation "d512 = d423"
equation "d514 = Plattenstärke"
equation "d515 = Plattenstärke"
equation "d516 = Plattenstärke"
equation "d517 = Plattenstärke / 2"
equation "d518 = Plattenstärke / 2"
equation "d519 = Plattenstärke / 2"
equation "d520 = Plattenstärke"
equation "d543 = Bohrung"
equation "d544 = Schraubenkopf"
equation "d545 = Bohrung"
equation "d546 = Schraubenkopf"
equation "d547 = Bohrung"
equation "d548 = Schraubenkopf"
equation "d550 = Bohrung"
equation "d551 = Schraubenkopf"
equation "d553 = Bohrung"
equation "d554 = Schraubenkopf"
equation "d555 = Bohrung"
equation "d556 = Schraubenkopf"
equation "d561 = Plattenstärke + Stützhöhe + 1.5 mm"
equation "d563 = ( Lochgröße - Kerblänge ) / 2"
equation "d564 = Kerblänge"
equation "d565 = Kerbtiefe"
equation "d566 = Lochgröße"
equation "d567 = Lochabstand"
equation "d568 = ( Lochgröße - Kerblänge ) / 2"
equation "d569 = Lochgröße"
equation "d570 = Lochabstand"
equation "d571 = Lochabstand"
equation "d572 = Lochgröße"
equation "d573 = -Kerbhöhe"
equation "d587 = Bohrung"
equation "d588 = Schraubenkopf"
equation "d589 = Bohrung"
equation "d590 = Schraubenkopf"
equation "d591 = Bohrung"
equation "d592 = Schraubenkopf"
equation "d593 = Bohrung"
equation "d594 = Schraubenkopf"
equation "d595 = Bohrung"
equation "d596 = Schraubenkopf"
equation "d597 = Bohrung"
equation "d598 = Schraubenkopf"
equation "d599 = Bohrung"
equation "d600 = Schraubenkopf"
equation "d601 = Bohrung"
equation "d602 = Schraubenkopf"
equation "d603 = Bohrung"
equation "d604 = Schraubenkopf"
equation "d605 = Bohrung"
equation "d606 = Schraubenkopf"
equation "d607 = Bohrung"
equation "d608 = Schraubenkopf"
equation "d609 = Bohrung"
equation "d610 = Schraubenkopf"
equation "d614 = ( Lochgröße - Kerblänge ) / 2"
equation "d621 = d620"
equation "d622 = Bohrung"
equation "d624 = Bohrung"
equation "d625 = Bohrung"
equation "d628 = 62.275 mm + 1.25 mm"
equation "d629 = 24.175 mm + 1.25 mm"
equation "d632 = Schraubenkopf"
equation "d633 = Schraubenkopf"
equation "d634 = d635 / 2"
equation "d637 = d636 / 2"
equation "d638 = ( Lochgröße - Kerblänge ) / 2"
equation "d639 = ( Lochgröße - Kerblänge ) / 2"
equation "d640 = ( Lochgröße - Kerblänge ) / 2"
equation "d641 = ( Lochgröße - Kerblänge ) / 2"
equation "d642 = ( Lochgröße - Kerblänge ) / 2"
equation "d643 = ( Lochgröße - Kerblänge ) / 2"
equation "d644 = ( Lochgröße - Kerblänge ) / 2"
equation "d645 = Gewinde"
equation "Gewinde = 2 mm"
equation "d649 = Gewinde"
equation "d651 = Gewinde"
equation "d653 = Gewinde"
equation "d655 = Gewinde"
equation "d657 = Gewinde"
equation "d659 = Plattenstärke + Stützhöhe"
equation "d661 = Gewinde"
equation "d662 = Gewinde"
equation "d663 = Gewinde"
equation "d664 = Gewinde"
equation "d665 = Gewinde"
equation "d666 = Gewinde"
equation "d667 = Gewinde"
equation "d668 = Gewinde"
equation "d669 = Gewinde"
equation "d670 = Gewinde"
equation "d671 = Gewinde"
equation "d672 = Gewinde"
equation "d676 = ( ( 6.75 - 3 ) / 2 ) * 1 mm"
equation "d679 = d676"
equation "d680 = d676"
equation "d681 = d676"
equation "d682 = d676"
equation "d683 = d676"
equation "d684 = d676"
equation "d685 = d676"
equation "d689 = ( Lochgröße - Kerblänge ) / 2"
equation "d690 = ( Lochgröße - Kerblänge ) / 2"
equation "d691 = d688"
equation "d692 = d687"
equation "d693 = d687"
equation "d694 = d688"
equation "d695 = ( Lochgröße - Kerblänge ) / 2"
equation "d696 = d687"
equation "d697 = d688"
equation "Stützhöhe = 8 mm"
equation "d705 = d548 + 2.5 mm"
equation "d706 = d551 + 2.5 mm"
equation "d707 = d544 + 2.5 mm"
equation "d708 = d546 + 2.5 mm"
equation "d709 = d556 + 2.5 mm"
equation "d710 = d554 + 2.5 mm"
equation "d711 = Plattenstärke + Stützhöhe"
named bodies: "Platte Rechts", "Bodenplatte Rechts", "Platte Mitte", "Rahmen Rechts", "Rahmen Mitte", "Bodenplatte Mitte", "Platte Links", "Bodenplatte Links", "Rahmen Links"
